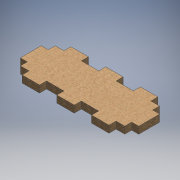
# Autodesk Inventor part: IBeamHorizantal
Saved by Autodesk Inventor 2016 (Build 200138000, 138)
## iProperties
Created: 2015-12-14
Part Number: IBeamHorizantal
Material: MDF Medium Density Fiberboard
Document SubType Name: Modeling
Designer: momem
Density: 0.8 g/cm^3
Appearance: Cardboard - Corrugated
Author: momem
Autodesk Inventor part; units mm, degrees
ref_plane "YZ Plane" through (0, 0, 0) normal (1, 0, 0) x (0, 1, 0)
ref_plane "XZ Plane" through (0, 0, 0) normal (0, 1, 0) x (-1, 0, 0)
ref_plane "XY Plane" through (0, 0, 0) normal (0, 0, 1) x (1, 0, 0)
sketch "Sketch1" plane through (0, 0, 0) normal (0, 0, 1) x (1, 0, 0)
  line L0 (14.2734, 15.7638) -> (14.2734, 22.1538)
  line L1 (14.2734, 22.1538) -> (30.0403, 22.1538)
  line L2 (30.0403, 22.1538) -> (30.0403, 15.7638)
  line L3 (14.2734, 15.7638) -> (6.39, 15.7638)
  line L4 (6.39, 15.7638) -> (6.39, 9.4794)
  line L5 (6.39, 9.4794) -> (0, 9.4794)
  line L6 (0, 9.4794) -> (0, -9.4794)
  line L7 (0, -9.4794) -> (6.39, -9.4794)
  line L8 (6.39, -9.4794) -> (6.39, -15.7638)
  line L9 (6.39, -15.7638) -> (14.2734, -15.7638)
  line L10 (45.8071, 22.1538) -> (61.574, 22.1538)
  line L11 (45.8071, 15.7638) -> (45.8071, 22.1538)
  line L12 (61.574, 22.1538) -> (61.574, 15.7638)
  line L13 (77.3409, 22.1538) -> (93.1077, 22.1538)
  line L14 (77.3409, 15.7638) -> (77.3409, 22.1538)
  line L15 (93.1077, 22.1538) -> (93.1077, 15.7638)
  line L16 (30.0403, 15.7638) -> (45.8071, 15.7638)
  line L17 (61.574, 15.7638) -> (77.3409, 15.7638)
  line L18 (0, 0) -> (107.3811, 0) construction
  line L19 (14.2734, -15.7638) -> (14.2734, -22.1538)
  line L20 (14.2734, -22.1538) -> (30.0403, -22.1538)
  line L21 (30.0403, -22.1538) -> (30.0403, -15.7638)
  line L22 (45.8071, -22.1538) -> (61.574, -22.1538)
  line L23 (45.8071, -15.7638) -> (45.8071, -22.1538)
  line L24 (61.574, -22.1538) -> (61.574, -15.7638)
  line L25 (77.3409, -22.1538) -> (93.1077, -22.1538)
  line L26 (77.3409, -15.7638) -> (77.3409, -22.1538)
  line L27 (93.1077, -22.1538) -> (93.1077, -15.7638)
  line L28 (30.0403, -15.7638) -> (45.8071, -15.7638)
  line L29 (61.574, -15.7638) -> (77.3409, -15.7638)
  line L30 (53.6906, 22.1538) -> (53.6906, -22.1538) construction
  line L31 (93.1077, 15.7638) -> (100.9911, 15.7638)
  line L32 (100.9911, 15.7638) -> (100.9911, 9.4794)
  line L33 (100.9911, 9.4794) -> (107.3811, 9.4794)
  line L34 (107.3811, 9.4794) -> (107.3811, -9.4794)
  line L35 (107.3811, -9.4794) -> (100.9911, -9.4794)
  line L36 (100.9911, -9.4794) -> (100.9911, -15.7638)
  line L37 (100.9911, -15.7638) -> (93.1077, -15.7638)
  line L38 (22.1569, 22.1538) -> (22.1569, -22.1538) construction
  dimension "d0" = 6.39
  dimension "d1" = 15.7669
  dimension "d4" = 31.5337
  dimension "d10" = 18.9588
  dimension "d11" = 31.5277
  dimension "d12" = 94.6011
  dimension "d13" = 6.39
  constraints: 78 end point, 18 symmetric about line, 7 perpendicular, 6 midpoint, 4 horizontal, 4 point on line, 2 collinear, 1 coincident, 1 vertical, 14 other
  measures "d0" distance of L0.start L0.end
  measures "d1" distance of L0.end L1.end
  measures "d4" distance of L0.end L10.start
  measures "d10" distance of L5.end L6.end
  measures "d11" distance between parallel lines of L9 L3
  measures "d12" distance between parallel lines of L32 L4
  measures "d13" distance of L4.end L5.end
extrude "Extrusion2" add sketch "Sketch1" along normal blind 6.39
equation "\"d0\" = WoodThickness"
equation "\"d1\" = 0.166667 * d7"
equation "\"d4\" = 0.333333 * d7"
equation "\"d10\" = 0.25 * DiskGap"
equation "\"d11\" = 0.5 * DiskGap - WoodThickness"
equation "\"d12\" = d7"
equation "\"d13\" = WoodThickness"
equation "\"d33\" = WoodThickness"
equation "\"WoodThickness\" = 6.39"
equation "\"d7\" = 94.601145"
equation "\"DiskGap\" = 75.835317"
body "Solid2"
